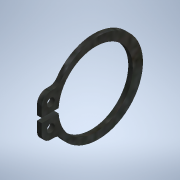
# Autodesk Inventor part: RRING-C-EXT-17
Saved by Autodesk Inventor 2021.3 (Build 253353000, 353)
## iProperties
Part Number: RRING-C-EXT-17
Material: Steel
Catalog Web Link: www.cadenas.de
Description: RRING_C_EXT-Retaining Rings - C (External) - JIS
Vendor: MISUMI
Document SubType Name: Modeling
Designer: partserver
Manufacturer: MISUMI
Mass: 0.865967 g
Surface Area: 3.53903 cm^2
Volume: 0.110314 cm^3
Density: 7.85 g/cm^3
Appearance: Plate
Category: PARTsolutions
Company: MISUMI
PSOL_IDENT_0: {$CADENAS_DATA\23d-libs\misumi\metric\accessories\rring_c_ext.prj},177 {VTYP=3D},{NB=RRING-C-EXT-17}
PSOL_IDENT_1: ,{LINA=RRING-C-EXT-17},{NN=RRING_C_EXT},{DATE=30.06.2021 13:30:10},{GEOMDATE=04.08.2015 01:36:13},{V
PSOL_IDENT_2: ERSION=},{LINEID=140},{WBVAR=MAT},{WBNUMERIC=}  {NB=RRING-C-EXT-17},{LINA=RRING-C-EXT-17},{KT=DUMMY}
PSOL_IDENT_3: ,{PN=RRING-C-EXT-17},{TYPE=RRING-C-EXT},{MAT= },{HARD=36~44HRC},{NO=17},{MATALG=' ','-','-S','304 St
PSOL_IDENT_4: ainless Steel-CSP'},{MATPN=},{DD3=15.7},{DD3TOL=+0.18/-0.18},{TT=1.00},{TTTOL=+0.05/-0.05},{BB=2.2},
PSOL_IDENT_5: {AA=3.7},{DD0=1.7},{DD4=25.0},{DD1=17},{DD2=16.20},{DD2TOL=0/-0.11},{MM=1.15},{MMTOL=+0.14/0},{NN=1.
PSOL_IDENT_6: 5},{H1=2},{A3=1.00},{A2=4.90},{A1=9.20},{R2=2.00},{R1=2.00}
NB: RRING-C-EXT-17
NN: 1.5
NT: Retaining Rings - C (External) - JIS
NBSYN: $PN.
LINA: RRING-C-EXT-17
CATALOG: Misumi
PN: RRING-C-EXT-17
MAT: -
HARD: 36~44HRC
NO: 17
DD3: 15.7
DD3TOL: +0.18/-0.18
TT: 1
TTTOL: +0.05/-0.05
BB: 2.2
AA: 3.7
DD0: 1.7
DD4: 25
DD1: 17
DD2: 16.2
DD2TOL: 0/-0.11
MM: 1.15
MMTOL: +0.14/0
SUPPLIER: MISUMI
ARTICLENO: RRING-C-EXT-17
BOMINFO: RRING-C-EXT-17
CREATOR: CADENAS GmbH
Title: RRING-C-EXT-17
Author: Cadenas PARTsolutions
Comments: Retaining Rings - C (External) - JIS
Autodesk Inventor part; units mm, degrees
sketch "Sketch_6" plane through (0, 0, 0) normal (1, 0, 0) x (0, 1, 0)
  arc A0 (-7.5166, -5.4766) -> (-7.5166, 5.4766) centre (0.55, 0) ccw
  arc A1 (-9.1712, 4.6) -> (-7.5166, 5.4766) centre (-9.1712, 6.6) ccw
  line L0 (-9.1712, 4.6) -> (-9.8, 4.6)
  arc A2 (-9.8, 4.6) -> (-11.8, 2.6) centre (-9.8, 2.6) ccw
  line L1 (-11.8, 2.6) -> (-11.8, 0.5)
  line L2 (-11.8, 0.5) -> (-8.0846, 0.5)
  arc A3 (-8.0846, -0.5) -> (-8.0846, 0.5) centre (0, 0) ccw
  line L3 (-8.0846, -0.5) -> (-11.8, -0.5)
  line L4 (-11.8, -0.5) -> (-11.8, -2.6)
  arc A4 (-11.8, -2.6) -> (-9.8, -4.6) centre (-9.8, -2.6) ccw
  line L5 (-9.8, -4.6) -> (-9.1712, -4.6)
  arc A5 (-7.5166, -5.4766) -> (-9.1712, -4.6) centre (-9.1712, -6.6) ccw
  circle A6 centre (-9.8, -2.45) radius 0.85
  circle A7 centre (-9.8, 2.45) radius 0.85
  constraints: 12 end point, 12 point on circle, 8 centre point
extrude "Extrusion1" add sketch "Sketch_6" along normal mid plane 1
ref_plane "1_XY" through (0, 0, 0) normal (1, 0, 0) x (0, 0, -1)
ref_plane "1_YZ" through (0, 0, 0) normal (0, 0, -1) x (0, 1, 0)
ref_plane "1_ZX" through (0, 0, 0) normal (0, 1, 0) x (1, 0, 0)
ref_plane "combination_module_XY" through (0.5, 0, 0) normal (1, 0, 0) x (0, 0, -1)
ref_plane "combination_module_YZ" through (0.5, 0, 0) normal (0, 0, -1) x (0, 1, 0)
ref_plane "combination_module_ZX" through (0.5, 0, 0) normal (0, 1, 0) x (1, 0, 0)
body "Solid1"
